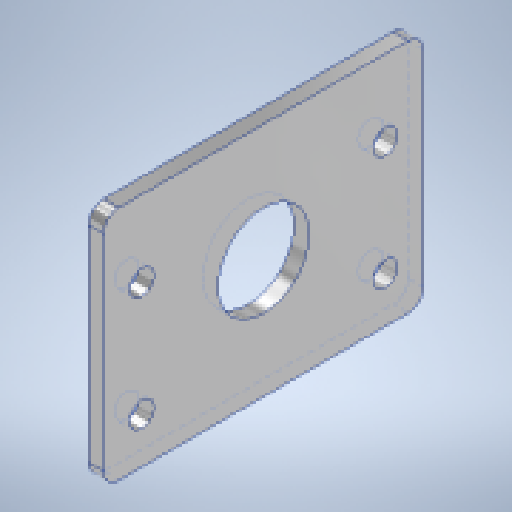
# Autodesk Inventor part: 2mm_double_for_pulley
Saved by Autodesk Inventor 2025 (Build 290162000, 162)
## iProperties
Created: 2025-02-24
Part Number: 2mm_double_for_pulley
Material: アルミニウム 6061
Document SubType Name: Modeling
Designer: Zhopa
Density: 2.7 g/cm^3
Appearance: アルミニウム - フラット
Mass: 6.22782 g
Surface Area: 27.4755 cm^2
Volume: 2.3066 cm^3
Author: Zhopa
Autodesk Inventor part; units mm, degrees
ref_plane "YZ Plane" through (0, 0, 0) normal (1, 0, 0) x (0, 1, 0)
ref_plane "XZ Plane" through (0, 0, 0) normal (0, 1, 0) x (-1, 0, 0)
ref_plane "XY Plane" through (0, 0, 0) normal (0, 0, 1) x (1, 0, 0)
sketch "Sketch1" plane through (0, 0, 0) normal (1, 0, 0) x (0, 1, 0)
  line L0 (-15.5, 21) -> (15.5, 21)
  line L1 (15.5, 21) -> (15.5, -21)
  line L2 (15.5, -21) -> (-15.5, -21)
  line L3 (-15.5, -21) -> (-15.5, 21)
  line L4 (-15.5, 21) -> (15.5, -21) construction
  line L5 (15.5, 21) -> (-15.5, -21) construction
  circle A0 centre (5.5, 16) radius 1.6
  circle A1 centre (5.5, -16) radius 1.6
  circle A2 centre (-9.5, -16) radius 1.6
  circle A3 centre (-9.5, 16) radius 1.6
  circle A4 centre (0, 0) radius 6
  point P0 (5.5, -16)
  point P1 (-9.5, -16)
  dimension "d0" = 42
  dimension "d1" = 31
  dimension "d2" = 5
  dimension "d3" = 10
  dimension "d5" = 15
  dimension "d6" = 5
  dimension "d7" = 3.2
  dimension "d8" = 3.2
  dimension "d9" = 3.2
  dimension "d10" = 3.2
  dimension "d11" = 12
  constraints: 12 end point, 5 centre point, 2 coincident, 2 midpoint, 2 parallel, 1 horizontal, 1 perpendicular
  measures "d0" distance of L0.end L1.end
  measures "d1" distance of L1.end L2.end
  measures "d2" distance from line of L0 point (5.5, 16)
  measures "d3" distance from line of point (5.5, 16) L1
  measures "d5" distance of point (5.5, 16) point (-9.5, 16)
  measures "d6" distance from line of L2 point (5.5, -16)
  measures "d7" diameter of A0
  measures "d8" diameter of A1
  measures "d9" diameter of A2
  measures "d10" diameter of A3
  measures "d11" diameter of A4
extrude "Extrusion1" add sketch "Sketch1" along normal blind 2
fillet "Fillet1" radius 2 4 edges at (1, 15.5, 21) (1, -15.5, 21) (1, -15.5, -21) (1, 15.5, -21)
body "Solid1"
